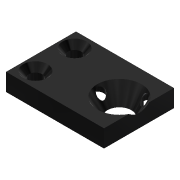
# Autodesk Inventor part: v2_bearing_insert_thick_three_point
Saved by Autodesk Inventor 2019 (Build 230136000, 136)
## iProperties
Created: 2017-04-27
Part Number: v2_bearing_insert_thick_three_point
Material: Acetal Resin, Black
Document SubType Name: Modeling
Designer: richp
Density: 1.425 g/cm^3
Appearance: Smooth - Black
Mass: 0.682972 g
Surface Area: 7.44256 cm^2
Volume: 0.479278 cm^3
bearing_thickness: 0.125 in
bb_diameter: 0.094 in
Author: richp
Autodesk Inventor part; units mm, degrees
sketch "Sketch1" plane through (0, 0, 0) normal (1, 0, 0) x (0, 1, 0)
  line L0 (-2.2715, 0) -> (9.3567, 0) construction
  line L1 (0, -10.9768) -> (0, 10.9768) construction
  line L2 (0, -1.7272) -> (0, -6.35)
  line L3 (0, -1.7272) -> (0, -1.7272)
  line L4 (0, -1.7272) -> (1.7709, -2.7496)
  line L5 (3.175, -3.5603) -> (3.175, -6.35)
  line L6 (3.175, -6.35) -> (0, -6.35)
  arc A0 (0.1834, 0) -> (1.7709, 2.7496) centre (3.3584, 0) ccw construction
  line L7 (2.5647, 7.8406) -> (4.1522, 7.8406) construction
  line L8 (4.1522, 7.8406) -> (4.1522, -7.8406) construction
  line L9 (4.1522, -7.8406) -> (2.5647, -7.8406) construction
  line L10 (2.5647, -7.8406) -> (2.5647, 7.8406) construction
  line L11 (2.5647, 7.8406) -> (4.1522, -7.8406) construction
  line L12 (4.1522, 7.8406) -> (2.5647, -7.8406) construction
  line L13 (0, 1.7272) -> (0, 6.35)
  line L14 (0, 1.7272) -> (0, 1.7272)
  line L15 (0, 1.7272) -> (3.175, 3.5603)
  line L16 (3.175, 3.5603) -> (3.175, 6.35)
  line L17 (3.175, 6.35) -> (0, 6.35)
  arc A1 (1.7709, 2.7496) -> (0.1834, 0) centre (3.3584, 0) ccw construction
  line L18 (1.7709, -2.7496) -> (3.175, -3.5603)
  line L19 (1.7709, 2.7496) -> (1.7709, -2.7496) construction
  point P0 (0, 0)
  point P1 (2.3851, -3.0222)
  point P2 (2.3851, 3.0222)
  dimension "d12" = 60
  dimension "d13" = 0
  dimension "bearing_thickness" = 3.175
  dimension "d15" = 1.7272
  dimension "d17" = 6.35
  dimension "d18" = 1.5875
  dimension "d23" = 12.7
  dimension "d52" = 3.3584
  constraints: 36 end point, 7 point on circle, 5 symmetric about line, 4 perpendicular, 4 point on line, 2 centre point, 2 horizontal, 2 midpoint, 2 parallel, 2 tangent, 1 coincident
  measures "d12" angle of L1 L4
  measures "d13" distance of L2.start L3.end
  measures "bearing_thickness" distance of L5.end L2.end
  measures "d15" distance from line of point (0, 0) L3
  measures "d17" diameter of A0
  measures "d18" distance between parallel lines of L10 L8
  measures "d23" distance between parallel lines of L6 L17
  measures "d52" distance from line of L2 A0.centre
sketch "Sketch11" plane through (0, 0, 0) normal (1, 0, 0) x (0, 1, 0)
  line L0 (3.175, 6.35) -> (0, 6.35) projected
  line L1 (3.175, -6.35) -> (0, -6.35) projected
  line L2 (-2.2715, 0) -> (9.3567, 0) construction
  line L3 (0, -10.9768) -> (0, 10.9768) construction
  line L4 (3.175, 6.35) -> (3.175, 0.762)
  line L5 (3.175, 0.762) -> (0, 0.762)
  line L6 (0, 6.35) -> (0, 0.762)
  line L7 (3.175, -6.35) -> (0, -6.35)
  line L8 (0, 10.9768) -> (0, -10.9768) construction
  line L9 (3.175, -6.35) -> (3.175, -0.762)
  line L10 (3.175, -0.762) -> (0, -0.762)
  line L11 (0, -6.35) -> (0, -0.762)
  point P0 (0, 0)
  dimension "d54" = 5.588
  constraints: 16 end point, 4 symmetric about line, 2 perpendicular, 2 point on line, 1 vertical
  measures "d54" distance of L0.start L4.end
extrude "Extrusion4" add sketch "Sketch11" along normal blind 3.556 and the other way blind 14.224
sketch "Sketch17" plane through (3.556, 0, 0) normal (1, 0, 0) x (0, 0, -1)
  line L0 (-6.35, 3.175) -> (-0.762, 3.175) projected
  line L1 (-0.762, 3.175) -> (0.762, 3.175)
  line L2 (0.762, 3.175) -> (0.762, 0)
  line L3 (0.762, 0) -> (-0.762, 0)
  line L4 (-0.762, 0) -> (-0.762, 3.175)
  point P0 (0, 0)
  constraints: 8 end point, 2 parallel, 1 horizontal, 1 perpendicular
ref_plane "Work Plane3" through (0, 3.175, 6.35) normal (1, 0, 0) x (0, -1, 0)
extrude "Extrusion6" add sketch "Sketch17" against normal blind 17.78
sketch "Sketch14" plane through (-14.224, 3.175, -6.35) normal (0, 1, 0) x (1, 0, 0)
  line L0 (-3.556, -6.35) -> (21.336, -6.35) projected
  line L1 (0, -5.588) -> (0, 0) projected
  point P0 (14.224, -6.35)
  point P1 (2.54, -2.794)
  point P2 (7.112, -2.794)
  point P3 (2.54, -9.906)
  point P4 (7.112, -9.906)
  dimension "d65" = 7.112
  dimension "d66" = 11.684
  dimension "d67" = 3.556
  constraints: 2 symmetric about line, 1 horizontal alignment
  measures "d65" horizontal distance of point (7.112, -2.794) point (14.224, -6.35)
  measures "d66" horizontal distance of point (2.54, -2.794) point (14.224, -6.35)
  measures "d67" distance from line of L0 point (2.54, -2.794)
hole "Hole2" at (-11.684, 3.175, -3.556) at (-11.684, 3.175, 3.556) direction (0, -1, 0) diameter 2.4384 depth 6.6294 tip angle 118 countersink diameter 4.3688 countersink angle 82 clearance for "Flat Head Machine Screw (82)" size "#2" standard "Ansi Unified Screw Threads"
sketch "Sketch12" plane through (0, 3.175, 6.35) normal (1, 0, 0) x (0, -1, 0)
  line L0 (3.175, 4.6228) -> (0, 2.7897) projected
  line L1 (3.175, 8.0772) -> (0, 9.9103) projected
  line L2 (5.4465, 6.35) -> (-6.1817, 6.35) construction
  line L3 (3.175, 17.3268) -> (3.175, -4.6268) construction
  line L4 (3.175, 4.6228) -> (3.175, 7.0113)
  line L5 (3.175, 4.6228) -> (3.175, 4.6228)
  line L6 (3.175, 8.0772) -> (3.175, 8.0772)
  line L7 (3.175, 7.0113) -> (3.175, 8.0772)
  line L8 (0, 2.7897) -> (0, 9.9103)
  line L9 (0, 0) -> (0, 5.588) projected
  point P0 (3.175, 6.35)
  constraints: 10 end point, 4 collinear, 3 point on line
extrude "Extrusion5" [suppressed]
ref_plane "Work Plane4" through (0, 2.5647, -7.8406) normal (-1, 0, 0) x (0, 0, 1)
sketch "Sketch16" plane through (0, 2.5647, -7.8406) normal (-1, 0, 0) x (0, 0, 1)
  line L0 (6.1134, -2.5647) -> (4.2803, 0.6103) projected
  line L1 (9.5678, -2.5647) -> (11.4008, 0.6103) projected
  line L2 (11.4008, 0.6103) -> (4.2803, 0.6103) projected
  line L3 (7.1793, -2.5647) -> (6.1134, -2.5647) projected
  line L4 (9.5678, -2.5647) -> (7.1793, -2.5647) projected
  line L5 (9.5678, -2.5647) -> (9.5678, -2.5647)
  line L6 (6.1134, -2.5647) -> (6.1134, -2.5647)
  line L7 (7.8406, -4.8362) -> (7.8406, 6.7921) projected
  line L8 (7.8406, 0.6103) -> (7.8406, -2.5647)
  constraints: 6 end point, 1 collinear, 1 midpoint, 1 point on line
revolve "Revolution7" cut sketch "Sketch16" angle 360 about axis through (0, 3.175, 0) along (0, -1, 0) contours L2 L1 L4 L7
sketch "Sketch22" plane through (0, 0, 0) normal (1, 0, 0) x (0, 1, 0)
  line L0 (0, -1.7272) -> (1.7709, -2.7496) projected
  line L1 (1.7709, -2.7496) -> (3.175, -3.5603) projected
  circle A0 centre (1.7304, -4.0507) radius 1.1906
  arc A1 (0.1834, 0) -> (1.7709, 2.7496) centre (3.3584, 0) ccw construction
  line L2 (1.8202, -2.8036) -> (2.1744, -2.946) construction
  line L3 (2.1744, -2.946) -> (0.782, -2.3864) construction
  line L4 (3.175, -3.5603) -> (3.175, -6.35) projected
  line L5 (0, -1.7272) -> (0, -6.35) projected
  line L6 (2.921, -4.0507) -> (2.921, -7.4115) construction
  point P0 (0, 0)
  dimension "d101" = 2.3813
  dimension "d102" = 0.254
  dimension "bb_drill_depth" = 2.921
  dimension "bb_mid_depth" = 1.7272
  constraints: 6 end point, 2 tangent, 2 vertical, 1 coincident, 1 horizontal alignment, 1 point on circle, 4 other
  measures "bb_drill_depth" distance between parallel lines of L6 L5
sketch "Sketch23" plane through (0, 0, 0) normal (0, 1, 0) x (-1, 0, 0)
  line L0 (0, -2.8601) -> (0, -5.2413) projected
  circle A0 centre (0, -4.0507) radius 1.1906 construction
  line L1 (0, 0) -> (3.8458, -3.8458) construction
  line L2 (0, -10.9768) -> (0, 10.9768) projected
  circle A1 centre (4.0507, 0) radius 1.1906
  line L3 (0, 0) -> (2.1149, 3.6631) construction
  line L4 (6.9328, 0) -> (-4.9074, 0) projected
  circle A2 centre (-2.0254, 3.508) radius 1.1906
  circle A3 centre (-2.0254, -3.508) radius 1.1906
  dimension "d88" = 45
  dimension "d89" = 60
  constraints: 4 end point, 3 centre point, 3 symmetric about line, 1 coincident, 1 vertical alignment, 5 other
  measures "d88" angle of L2 L1
  measures "d89" angle of L3 L4
extrude "Extrusion9" cut sketch "Sketch23" along normal blind 1.7272
ref_plane "Work Plane9" through (0, 1.7304, -4.0507) normal (0, 1, 0) x (-1, 0, 0)
sketch "Sketch25" plane through (0, 0, 0) normal (1, 0, 0) x (0, 1, 0)
  line L0 (0, 1.7272) -> (3.175, 3.5603) projected
  line L1 (0, -1.7272) -> (1.7709, -2.7496) projected
  line L2 (1.7709, -2.7496) -> (3.175, -3.5603) projected
  line L3 (0, 2.1671) -> (3.175, 4.0002)
  line L4 (3.175, 3.5603) -> (3.175, -3.5603)
  line L5 (3.175, 3.5603) -> (3.175, 4.0002)
  line L6 (0, 1.7272) -> (0, 2.1671)
  line L7 (0, 1.7272) -> (0, -1.7272)
  line L8 (-2.2715, 0) -> (9.3567, 0) projected
  line L9 (0, -2.1671) -> (3.175, -4.0002)
  line L10 (3.175, -3.5603) -> (3.175, -4.0002)
  line L11 (0, -1.7272) -> (0, -2.1671)
  point P0 (0, 0)
  point P1 (0, 0)
  dimension "d95" = 0.381
  constraints: 16 end point, 4 vertical, 2 symmetric about line, 1 parallel, 1 point on line
  measures "d95" distance between parallel lines of L0 L3
revolve "Revolution11" cut sketch "Sketch25" angle 360 about axis through (0, -10, 0) along (0, 1, 0) contours L6 L3 L5 L0
sketch "Sketch24" plane through (0, 1.7304, -4.0507) normal (0, 1, 0) x (-1, 0, 0)
  circle A0 centre (4.0507, 4.0507) radius 1.1906 projected
  circle A1 centre (-2.0254, 7.5587) radius 1.1906 projected
  circle A2 centre (-2.0254, 0.5427) radius 1.1906 projected
  line L0 (-2.0254, 7.5587) -> (-2.0254, 6.3681)
  line L1 (-2.0254, 7.5587) -> (-2.0254, 8.7493)
  line L2 (-2.0254, 0.5427) -> (-2.0254, 1.7333)
  line L3 (-2.0254, 0.5427) -> (-2.0254, -0.6479)
  line L4 (4.0507, 4.0507) -> (4.0507, 5.2413)
  line L5 (4.0507, 4.0507) -> (4.0507, 2.8601)
  point P0 (0, 4.0507)
  constraints: 12 end point, 6 point on circle, 3 vertical, 2 point on line, 1 parallel
revolve "Revolution8" cut sketch "Sketch24" angle 360 about axis through (-4.0507, 1.7304, 0) along (0, 0, 1) picked at (3.9557, 3.2685) contours L4 L5 A0
revolve "Revolution9" cut sketch "Sketch24" angle 360 about axis through (2.0254, 1.7304, 3.508) along (0, 0, 1) picked at (-2.1204, 6.7765) contours L1 L0 A1
revolve "Revolution10" cut sketch "Sketch24" angle 360 about axis through (2.0254, 1.7304, -3.508) along (0, 0, 1) picked at (-2.1204, -0.2395) contours L2 L3 A2
sketch "Sketch26" plane through (-14.224, 0, 6.35) normal (0, -1, 0) x (1, 0, 0)
  line L0 (10.1733, -6.35) -> (0, -6.35) construction
  line L1 (0, 0) -> (0, -12.7) construction
  line L2 (7.112, -9.906) -> (7.112, -2.794) construction
  line L3 (8.3026, -9.906) -> (8.3026, -8.3344)
  line L4 (5.9214, -2.794) -> (5.9214, -4.3656)
  arc A0 (5.9214, -9.906) -> (7.112, -11.0966) centre (7.112, -9.906) ccw
  arc A1 (8.3026, -2.794) -> (7.112, -1.6034) centre (7.112, -2.794) ccw
  line L5 (5.9214, -4.3656) -> (5.9214, -8.3344)
  line L6 (5.9214, -8.3344) -> (5.9214, -9.906)
  line L7 (8.3026, -8.3344) -> (8.3026, -2.794)
  circle A2 centre (7.112, -2.794) radius 1.2192 projected
  circle A3 centre (16.2494, -2.842) radius 1.1906 projected
  line L8 (7.112, -1.6034) -> (11.1812, -1.6034)
  arc A4 (17.1818, -3.5824) -> (16.2494, -2.842) centre (14.224, -6.35) ccw construction
  circle A5 centre (10.1733, -6.35) radius 1.1906 projected
  arc A6 (17.0431, -1.4672) -> (11.1812, -1.6034) centre (14.224, -6.35) ccw
  line L9 (16.2494, -2.842) -> (17.0431, -1.4672)
  line L10 (16.2494, -9.858) -> (17.0431, -11.2328)
  arc A7 (16.2494, -9.858) -> (17.1818, -3.5824) centre (14.224, -6.35) ccw construction
  arc A8 (16.2494, -2.842) -> (16.2494, -9.858) centre (14.224, -6.35) ccw
  circle A9 centre (7.112, -9.906) radius 1.2192 projected
  arc A10 (11.1812, -1.6034) -> (11.1812, -11.0966) centre (14.224, -6.35) ccw
  arc A11 (11.1812, -11.0966) -> (17.0431, -11.2328) centre (14.224, -6.35) ccw
  arc A12 (7.112, -11.0966) -> (8.3026, -9.906) centre (7.112, -9.906) ccw
  arc A13 (7.112, -1.6034) -> (5.9214, -2.794) centre (7.112, -2.794) ccw
  line L11 (11.1812, -11.0966) -> (7.112, -11.0966)
  point P0 (16.2494, -2.842)
  point P1 (9.3701, -8.5295)
  point P2 (7.112, -6.35)
  point P3 (8.3026, -4.3656)
  dimension "d106" = 2.3813
  dimension "d110" = 1.5875
  constraints: 24 end point, 24 point on circle, 23 tangent, 10 centre point, 5 parallel, 4 point on line, 2 coincident, 2 horizontal, 2 line through centre, 2 midpoint, 2 symmetric about line, 1 vertical, 3 other
  measures "d106" diameter of A1
  measures "d110" radial gap between concentric circles of A6 A4
extrude "Extrusion11" [suppressed]
sketch "Sketch27" plane through (-14.224, 0, 6.35) normal (0, -1, 0) x (1, 0, 0)
  circle A0 centre (16.2494, -9.858) radius 1.1906 projected
  circle A1 centre (16.2494, -2.842) radius 1.1906 projected
  circle A2 centre (10.1733, -6.35) radius 1.1906 construction
  circle A3 centre (7.112, -9.906) radius 1.2192 construction
  circle A4 centre (7.112, -2.794) radius 1.2192 construction
  line L0 (5.8928, -9.906) -> (5.8928, -9.5377) construction
  arc A5 (16.8447, -1.8109) -> (12.0632, -1.5748) centre (14.224, -6.35) ccw
  arc A6 (16.8866, -3.8477) -> (15.0597, -2.793) centre (14.224, -6.35) ccw construction
  line L1 (7.4803, -11.1252) -> (12.0632, -11.1252)
  line L2 (7.112, -1.5748) -> (7.4803, -1.5748) construction
  arc A7 (16.8447, -10.8891) -> (16.8447, -1.8109) centre (14.224, -6.35) ccw construction
  arc A8 (16.8866, -8.8523) -> (16.8866, -3.8477) centre (14.224, -6.35) ccw construction
  arc A9 (15.0597, -2.793) -> (15.0597, -9.907) centre (14.224, -6.35) ccw
  arc A10 (15.0597, -9.907) -> (16.8866, -8.8523) centre (14.224, -6.35) ccw construction
  arc A11 (15.0597, -9.907) -> (16.8447, -10.8891) centre (16.2494, -9.858) ccw
  arc A12 (16.8447, -1.8109) -> (15.0597, -2.793) centre (16.2494, -2.842) ccw
  arc A13 (12.0632, -11.1252) -> (16.8447, -10.8891) centre (14.224, -6.35) ccw
  arc A14 (12.0632, -1.5748) -> (12.0632, -11.1252) centre (14.224, -6.35) ccw construction
  line L3 (7.112, -11.1252) -> (7.4803, -11.1252) construction
  line L4 (5.8928, -9.906) -> (5.8928, -9.5377) construction
  line L5 (5.8928, -2.794) -> (5.8928, -3.1623) construction
  line L6 (7.112, -1.5748) -> (7.4803, -1.5748) construction
  arc A15 (5.8928, -9.5377) -> (7.4803, -11.1252) centre (7.4803, -9.5377) ccw
  arc A16 (7.4803, -1.5748) -> (5.8928, -3.1623) centre (7.4803, -3.1623) ccw
  line L7 (5.8928, -9.5377) -> (5.8928, -3.1623)
  line L8 (7.4803, -1.5748) -> (12.0632, -1.5748)
  dimension "d114" = 1.5875
  dimension "d124" = 1.5875
  constraints: 35 point on circle, 18 end point, 12 centre point, 12 tangent, 4 coincident, 4 horizontal, 3 vertical, 1 equal radius, 1 perpendicular
  measures "d114" radial gap between concentric circles of A5 A6
  measures "d124" radius of A15
extrude "Extrusion13" cut sketch "Sketch27" along normal mid plane 2.286 contours A0 A13 L1 A15 L7 A16 L8 A5 A1 A9
equation "\"d15\" = bearing_spacing"
equation "\"d65\" = hole1_setback"
equation "\"d66\" = hole2_setback"
equation "\"d67\" = hole_lateral"
equation "\"d90\" = bb_mid_depth"
equation "\"d12\" = bearing_angle"
equation "\"d101\" = bb_diameter"
equation "\"hole1_setback_qq\" = 7.112"
equation "\"hole_lateral_qq\" = 3.556"
equation "\"hole2_setback_qq\" = 11.684"
equation "\"bearing_angle_qq\" = 60deg"
equation "\"bearing_spacing_qq\" = 1.7272"
equation "\"bb_diameter\" = 2.38125"
equation "\"bearing_angle\" = 60deg"
equation "\"bearing_spacing\" = 1.7272"
equation "\"hole1_setback\" = 7.112"
equation "\"hole2_setback\" = 11.684"
equation "\"hole_lateral\" = 3.556"
body "Solid2"
